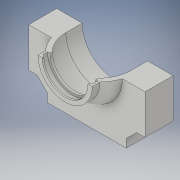
# Autodesk Inventor part: 20_Cube_Insert_Eye_Lens_v3
Saved by Autodesk Inventor 2019 (Build 230136000, 136)
## iProperties
Created: 2020-02-04
Part Number: 20_Cube_Insert_Eye_Lens_v3
Material: Generic
Document SubType Name: Modeling
Designer: marsikovabarbora
Density: 1 g/cm^3
Appearance: Default
Author: marsikovabarbora
Autodesk Inventor part; units mm, degrees
ref_plane "YZ Plane" through (0, 0, 0) normal (1, 0, 0) x (0, 1, 0)
ref_plane "XZ Plane" through (0, 0, 0) normal (0, 1, 0) x (-1, 0, 0)
sketch "Sketch1" plane through (0, 0, 0) normal (0, 0, 1) x (1, 0, 0)
  line L0 (-36.8533, 0) -> (46.8153, 0) construction
  line L1 (0, -29.8808) -> (0, 4.9801) construction
  line L2 (0, 0) -> (24.6516, -24.6516) construction
  line L3 (0, 0) -> (34.8626, 0) construction
  line L4 (0, -24.9006) -> (16.8, -24.9006)
  line L5 (16.8, -24.9006) -> (16.8, -21.2406)
  line L6 (16.8, -21.2406) -> (19.0203, -19.0203)
  line L7 (24.9006, 0) -> (24.9006, -16.8)
  line L8 (24.9006, -16.8) -> (21.2406, -16.8)
  line L9 (21.2406, -16.8) -> (19.0203, -19.0203)
  line L10 (0, 0) -> (-24.6516, -24.6516) construction
  line L11 (0, -24.9006) -> (-16.8, -24.9006)
  line L12 (-16.8, -24.9006) -> (-16.8, -21.2406)
  line L13 (-16.8, -21.2406) -> (-19.0203, -19.0203)
  line L14 (-24.9006, 0) -> (-24.9006, -16.8)
  line L15 (-24.9006, -16.8) -> (-21.2406, -16.8)
  line L16 (-21.2406, -16.8) -> (-19.0203, -19.0203)
  arc A0 (-14, 0) -> (14, 0) centre (0, 0) ccw
  line L17 (0, 0) -> (14, 0) construction
  line L18 (0, 0) -> (-14, 0) construction
  line L19 (-14, 0) -> (-24.9006, 0)
  line L20 (14, 0) -> (24.9006, 0)
  dimension "d0" = 45
  dimension "d1" = 16.8
  dimension "d2" = 3.66
  dimension "d4" = 3.14
  dimension "d5" = 14
  dimension "d6" = 180
  constraints: 38 end point, 10 symmetric about line, 4 point on line, 2 horizontal, 2 perpendicular, 2 point on circle, 1 centre point, 1 coincident, 1 equal length
  measures "d0" angle of L2 L3
  measures "d1" distance of L4.start L4.end
  measures "d2" distance of L4.end L5.end
  measures "d4" distance of L5.end L6.end
  measures "d5" radius of A0
  measures "d6" angle of L18 L17
extrude "Extrusion1" add sketch "Sketch1" along normal blind 5
sketch "Sketch3" plane through (-24.9006, 0, 0) normal (0, 1, 0) x (1, 0, 0)
  line L0 (10.9006, 0) -> (0, 0) construction
  line L1 (0, 0) -> (0, -5) construction
  line L2 (10.9006, -5) -> (0, -5) construction
  line L3 (10.9006, 0) -> (10.9006, -5) construction
  line L4 (38.9006, 0) -> (10.9006, 0) construction
  line L5 (10.9006, 0) -> (10.9006, -5) construction
  line L6 (38.9006, -5) -> (10.9006, -5) construction
  line L7 (38.9006, 0) -> (38.9006, -5) construction
  line L8 (49.8013, 0) -> (38.9006, 0) construction
  line L9 (38.9006, 0) -> (38.9006, -5) construction
  line L10 (49.8013, -5) -> (38.9006, -5) construction
  line L11 (49.8013, 0) -> (49.8013, -5) construction
  line L12 (24.9006, 18.5006) -> (24.9006, -23.5037) construction
  arc A0 (10.9006, 0) -> (24.9006, -14) centre (24.9006, 0) ccw
  arc A1 (8.9006, 0) -> (24.9006, -16) centre (24.9006, 0) ccw
  line L13 (24.9006, -16) -> (24.9006, -14)
  line L14 (10.9006, 0) -> (0, 0) projected
  line L15 (8.9006, 0) -> (10.9006, 0)
  dimension "d11" = 2
  constraints: 4 end point, 4 point on circle, 2 centre point, 1 coincident, 1 collinear, 1 horizontal, 1 point on line
  measures "d11" radial gap between concentric circles of A0 A1
revolve "Revolution2" add sketch "Sketch3" angle 180 about axis through (0, 0, -10) along (0, 0, 1)
ref_plane "Work Plane1" through (0, 0, 16) normal (0, 0, 1) x (1, 0, 0)
sketch "Sketch5" plane through (24.9006, 0, 5) normal (0, 1, 0) x (1, 0, 0)
  line L0 (0, 0) -> (-9.7019, 0) construction
  line L1 (0, 5) -> (0, 0) construction
  line L2 (0, 5) -> (-10.9006, 5) construction
  arc A0 (-38.9006, 5) -> (-10.9006, 5) centre (-24.9006, 5) ccw construction
  line L3 (-38.9006, 5) -> (-49.8013, 5) construction
  line L4 (-49.8013, 5) -> (-49.8013, 0) construction
  line L5 (-40.0993, 0) -> (-49.8013, 0) construction
  arc A1 (-40.0993, 0) -> (-9.7019, 0) centre (-24.9006, 5) ccw construction
  arc A2 (-38.9006, 5) -> (-10.9006, 5) centre (-24.9006, 5) ccw construction
  line L6 (-10.9006, 5) -> (-38.9006, 5) construction
  line L7 (-24.9006, 25) -> (-24.9006, -17) construction
  line L8 (-24.9006, -6) -> (-35.7006, -6)
  line L9 (-35.7006, -6) -> (-35.7006, -8.1)
  line L10 (-35.7006, -8.1) -> (-24.9006, -8.1)
  line L11 (-24.9006, -8.1) -> (-24.9006, -6)
  arc A3 (-10.9006, 5) -> (-38.9006, 5) centre (-24.9006, 5) ccw construction
  line L12 (-24.9006, 19) -> (-24.9006, -6) construction
  line L13 (-24.9006, 19) -> (0.0994, 19) construction
  line L14 (-34.7006, -6) -> (-33.5609, -6)
  line L15 (-33.5609, -6) -> (-33.5609, -4.998)
  line L16 (-33.5609, -4.998) -> (-34.7006, -4.998)
  line L17 (-34.7006, -4.998) -> (-34.7006, -6)
  arc A4 (-38.9006, 5) -> (-10.9006, 5) centre (-24.9006, 5) ccw projected
  line L18 (-24.9006, -8.1) -> (-34.087, -8.1)
  line L19 (-34.087, -8.1) -> (-34.087, -11)
  line L20 (-34.087, -11) -> (-24.9006, -11)
  line L21 (-24.9006, -11) -> (-24.9006, -8.1)
  arc A5 (-40.0993, 0) -> (-9.7019, 0) centre (-24.9006, 5) ccw projected
  dimension "d16" = 10.8
  dimension "d17" = 2.1
  dimension "d19" = 25
  dimension "d20" = 90
  dimension "d21" = 1
  constraints: 28 end point, 7 point on circle, 6 parallel, 4 horizontal, 4 perpendicular, 3 point on line, 1 centre point, 1 collinear, 1 other
  measures "d16" distance of L8.start L8.end
  measures "d17" distance of L8.end L9.end
  measures "d19" distance of L12.start L12.end
  measures "d20" angle of L12 L13
  measures "d21" distance between parallel lines of L9 L17
revolve "Revolution3" cut sketch "Sketch5" angle 360 about axis through (0, 0, -10) along (0, 0, 1) contours L11 L10 A4 L8 | A4 L10 A5 L9 L8 | L8 L17 A4 | L21 A4 L10 | A4 L21 A5 L10 | L10 L9 A5
sketch "Sketch6" plane through (-24.9006, 0, 5) normal (0, 1, 0) x (1, 0, 0)
  line L0 (14.1006, -6.8051) -> (14.1006, -6) construction
  line L1 (14.1006, -6) -> (15.1006, -6) construction
  line L2 (15.1006, -6) -> (15.1006, -4.998) construction
  arc A0 (10.9006, 5) -> (15.1006, -4.998) centre (24.9006, 5) ccw construction
  line L3 (10.9006, 5) -> (0, 5) construction
  line L4 (0, 5) -> (0, 0) construction
  line L5 (9.7019, 0) -> (0, 0) construction
  arc A1 (9.7019, 0) -> (14.1006, -6.8051) centre (24.9006, 5) ccw construction
  line L6 (24.9006, 7.4176) -> (24.9006, -9.5058) construction
  arc A2 (9.7019, 0) -> (14.1006, -6.8051) centre (24.9006, 5) ccw projected
  line L7 (13.2817, -6) -> (13.2817, -9.314)
  line L8 (14.1006, -6) -> (24.9006, -6) construction
  line L9 (24.9006, -6) -> (24.9006, -8) construction
  line L10 (24.9006, -8) -> (14.1006, -8) construction
  line L11 (14.1006, -8) -> (14.1006, -6) construction
  line L12 (35.7006, -6) -> (14.1006, -6) construction
  line L13 (14.1006, -6) -> (24.9006, -6) construction
  line L14 (24.9006, -6) -> (24.9006, -11.2) construction
  line L15 (24.9006, -11.2) -> (14.1006, -11.2) construction
  line L16 (14.1006, -11.2) -> (14.1006, -6) construction
  arc A3 (14.1006, -8) -> (24.9006, -11.2) centre (24.9006, 8.625) ccw construction
  line L17 (14.1006, -6.8051) -> (14.1006, -8)
  line L18 (13.2817, -9.314) -> (15.1006, -9.314)
  line L19 (15.1006, -9.314) -> (15.1006, -8.6084)
  line L20 (15.1006, -8.6084) -> (14.1006, -8)
  line L21 (13.2817, -6) -> (14.1006, -6)
  line L22 (35.7006, -6.8051) -> (14.1006, -6.8051) projected
  line L23 (14.1006, -6.8051) -> (14.1006, -6)
  dimension "d23" = 2
  dimension "d24" = 5.2
  constraints: 30 end point, 4 horizontal, 4 parallel, 4 perpendicular, 4 point on circle, 2 point on line, 1 centre point, 1 collinear, 1 tangent, 1 vertical
  measures "d23" distance of L10.end L0.end
  measures "d24" distance of L15.end L0.end
revolve "Revolution4" add sketch "Sketch6" angle 180 about axis through (0, 0, -10) along (0, 0, 1) contours A2 L17 L20 L19 L18 L7
sketch "Sketch7" plane through (0, 0, 0) normal (0, 0, -1) x (-1, 0, 0)
  line L0 (-24.9006, 0) -> (-14, 0) projected
  line L1 (-24.9006, -16.8) -> (-24.9006, 0) projected
  line L2 (-21.2406, -16.8) -> (-24.9006, -16.8) projected
  line L3 (-16.8, -21.2406) -> (-21.2406, -16.8) projected
  line L4 (-16.8, -24.9006) -> (-16.8, -21.2406) projected
  line L5 (16.8, -24.9006) -> (-16.8, -24.9006) projected
  line L6 (16.8, -21.2406) -> (16.8, -24.9006) projected
  line L7 (21.2406, -16.8) -> (16.8, -21.2406) projected
  line L8 (24.9006, -16.8) -> (21.2406, -16.8) projected
  line L9 (24.9006, 0) -> (24.9006, -16.8) projected
  line L10 (14, 0) -> (24.9006, 0) projected
  arc A0 (-14, 0) -> (14, 0) centre (0, 0) ccw projected
extrude "Extrusion3" add sketch "Sketch7" along normal blind 7
sketch "Skizze8" plane through (0, 0, 5) normal (0, 0, 1) x (1, 0, 0)
  arc A0 (-15.1987, 0) -> (15.1987, 0) centre (0, 0) ccw construction
  line L0 (-15.1987, 0) -> (-24.9006, 0) construction
  line L1 (-24.9006, 0) -> (-24.9006, -16.8) construction
  line L2 (-24.9006, -16.8) -> (-21.2406, -16.8) projected
  line L3 (-21.2406, -16.8) -> (-16.8, -21.2406) projected
  line L4 (-16.8, -21.2406) -> (-16.8, -24.9006) projected
  line L5 (-16.8, -24.9006) -> (16.8, -24.9006) construction
  line L6 (16.8, -24.9006) -> (16.8, -21.2406) projected
  line L7 (16.8, -21.2406) -> (21.2406, -16.8) projected
  line L8 (21.2406, -16.8) -> (24.9006, -16.8) projected
  line L9 (24.9006, -16.8) -> (24.9006, 0) construction
  line L10 (24.9006, 0) -> (15.1987, 0) construction
  line L11 (25.0006, 0.1) -> (25.0006, -16.9) construction
  line L12 (25.0006, -16.9) -> (21.2821, -16.9)
  line L13 (21.2821, -16.9) -> (16.9, -21.2821)
  line L14 (16.9, -21.2821) -> (16.9, -25.0006)
  line L15 (16.9, -25.0006) -> (-16.9, -25.0006) construction
  line L16 (-16.9, -25.0006) -> (-16.9, -21.2821)
  line L17 (-16.9, -21.2821) -> (-21.2821, -16.9)
  line L18 (-21.2821, -16.9) -> (-25.0006, -16.9)
  line L19 (-25.0006, -16.9) -> (-25.0006, 0.1) construction
  line L20 (-25.0006, 0.1) -> (-15.0984, 0.1) construction
  arc A1 (-15.0984, 0.1) -> (15.0984, 0.1) centre (0, 0) ccw construction
  line L21 (15.0984, 0.1) -> (25.0006, 0.1) construction
  line L22 (-24.9006, -16.8) -> (-24.9006, -16.9)
  line L23 (-16.8, -24.9006) -> (-16.9, -24.9006)
  line L24 (16.8, -24.9006) -> (-16.8, -24.9006) projected
  line L25 (16.8, -24.9006) -> (16.9, -24.9006)
  line L26 (24.9006, 0) -> (24.9006, -16.8) projected
  line L27 (24.9006, -16.8) -> (24.9006, -16.9)
  point P0 (0, 0)
  dimension "d0" = 45
  dimension "d1" = 16.8
  dimension "d2" = 3.66
  dimension "d4" = 3.14
  dimension "d5" = 14
  dimension "d6" = 180
  dimension "d28" = 0.1
  constraints: 30 end point, 5 point on line, 3 perpendicular, 2 point on circle, 1 centre point, 11 other
  measures "d28" distance between parallel lines of L9 L11
extrude "IM_offset" add sketch "Skizze8" against normal up to surface (12 mm away)
body "Solid1"
